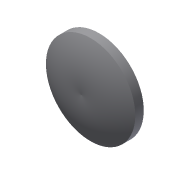
# Autodesk Inventor part: 00_Lens_f_29_d12.6
Saved by Autodesk Inventor 2019 (Build 230136000, 136)
## iProperties
Created: 2019-08-29
Part Number: 00_Lens_f_29_d12.6
Material: Generic
Document SubType Name: Modeling
Designer: diederichbenedict
Density: 1 g/cm^3
Appearance: Default
Author: diederichbenedict
Autodesk Inventor part; units mm, degrees
ref_plane "YZ Plane" through (0, 0, 0) normal (1, 0, 0) x (0, 1, 0)
ref_plane "XZ Plane" through (0, 0, 0) normal (0, 1, 0) x (-1, 0, 0)
ref_plane "XY Plane" through (0, 0, 0) normal (0, 0, 1) x (1, 0, 0)
sketch "Sketch1" plane through (0, 0, 0) normal (1, 0, 0) x (0, 1, 0)
  line L0 (0, 0) -> (6.3, 0)
  line L1 (6.3, 0) -> (6.3, 1.2)
  arc A0 (6.3, 1.2) -> (0, 2.5) centre (1.1584, -7.8017) ccw
  line L2 (0, 0) -> (0, 2.5)
  dimension "d0" = 6.3
  dimension "d1" = 1.2
  dimension "d2" = 2.5
  constraints: 6 end point, 2 point on circle, 1 centre point, 1 horizontal, 1 perpendicular
  measures "d0" distance of L0.start L0.end
  measures "d1" distance of L0.end L1.end
  measures "d2" distance from line of L2.end L0
revolve "Revolution1" add sketch "Sketch1" angle 360 about axis through (0, 0, 0) along (0, 0, 1)
body "Solid1"
